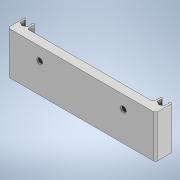
# Autodesk Inventor part: switch_mount
Saved by Autodesk Inventor 2020 (Build 240168000, 168)
## iProperties
Created: 2020-06-05
Part Number: switch_mount
Material: Generic
Document SubType Name: Modeling
Designer: suhren
Density: 1 g/cm^3
Appearance: Default
Author: suhren
Autodesk Inventor part; units mm, degrees
ref_plane "YZ Plane" through (0, 0, 0) normal (1, 0, 0) x (0, 1, 0)
ref_plane "XZ Plane" through (0, 0, 0) normal (0, 1, 0) x (-1, 0, 0)
ref_plane "XY Plane" through (0, 0, 0) normal (0, 0, 1) x (1, 0, 0)
sketch "Sketch1" plane through (0, 0, 0) normal (0, 1, 0) x (-1, 0, 0)
  line L0 (51.25, 0) -> (-51.25, 0)
  line L1 (-51.25, 0) -> (-51.25, 4.75)
  line L2 (-51.25, 6) -> (51.25, 6) construction
  line L3 (51.25, 6) -> (51.25, 4.75) construction
  line L4 (50, 6) -> (-50, 6)
  line L5 (-50, 6) -> (-51.25, 4.75)
  line L6 (50, 6) -> (51.25, 4.75)
  line L7 (51.25, 4.75) -> (51.25, 0)
  line L8 (-51.25, 4.75) -> (-51.25, 6) construction
  line L9 (47.5, -5.889) -> (44.95, -4.4167)
  line L10 (44.95, -4.4167) -> (44.95, -1.4722)
  line L11 (44.95, -1.4722) -> (47.5, 0)
  line L12 (47.5, 0) -> (50.05, -1.4722)
  line L13 (50.05, -1.4722) -> (50.05, -4.4167)
  line L14 (50.05, -4.4167) -> (47.5, -5.889)
  line L15 (47.5, -2.9445) -> (-47.5, -2.9445) construction
  line L16 (51.25, 0) -> (51.25, -5.0477)
  line L17 (51.25, -5.0477) -> (50.65, -5.6477)
  line L18 (50.65, -5.6477) -> (49.65, -4.6477)
  line L19 (50.05, -2.9445) -> (51.25, -2.9445) construction
  line L20 (45.35, -4.6477) -> (44.35, -5.6477)
  line L21 (44.35, -5.6477) -> (43.75, -5.0477)
  line L22 (43.75, -5.0477) -> (43.75, 0)
  line L23 (47.5, -5.889) -> (47.5, 0) construction
  line L24 (43.75, 0) -> (51.25, 0) construction
  point P0 (0, 0)
  point P1 (0, 0)
  point P2 (0, 0)
  point P3 (0, 6)
  point P4 (0, 6)
  point P5 (0, -2.9445)
  point P6 (50.65, -2.9445)
  dimension "d22" = 100
  dimension "d23" = 6
  dimension "d24" = 95
  dimension "d25" = 5.1
  dimension "d26" = 6
  dimension "d27" = 1.2
  dimension "d28" = 0.4
  constraints: 51 end point, 7 perpendicular, 7 point on line, 6 midpoint, 5 coincident, 5 parallel, 3 vertical, 2 horizontal, 2 horizontal alignment, 2 vertical alignment, 1 collinear, 16 other
  measures "d22" distance of L4.start L4.end
  measures "d23" distance between parallel lines of L0 L2
  measures "d24" distance of L15.end L15.start
  measures "d25" distance between parallel lines of L10 L13
  measures "d26" vertical distance of L2.end L11.end
  measures "d27" distance of L19.start L19.end
  measures "d28" horizontal distance of L18.end L13.end
extrude "Extrusion1" add sketch "Sketch1" along normal blind 29.5 contours L0 L1 L5 L4 L6 L7
extrude "Extrusion3" add sketch "Sketch1" along normal blind 29.5 contours L16 L17 L18 L14 L13 L12 L0 | L11 L10 L9 L20 L21 L22 L0
mirror "Mirror1" about plane through (0, 0, 0) normal (1, 0, 0) of "Extrusion3"
sketch "Sketch2" plane through (41.9, 0, 0) normal (0, 0, -1) x (-1, 0, 0)
  line L0 (41.9, 29.5) -> (41.9, 0) construction
  line L1 (12.9, 20.5) -> (70.9, 20.5) construction
  line L2 (9.35, 22.5496) -> (12.9, 24.5992)
  line L3 (12.9, 24.5992) -> (16.45, 22.5496)
  line L4 (16.45, 22.5496) -> (16.45, 18.4504)
  line L5 (16.45, 18.4504) -> (12.9, 16.4008)
  line L6 (12.9, 16.4008) -> (9.35, 18.4504)
  line L7 (9.35, 18.4504) -> (9.35, 22.5496)
  line L8 (74.45, 22.5496) -> (74.45, 18.4504)
  line L9 (74.45, 18.4504) -> (70.9, 16.4008)
  line L10 (70.9, 16.4008) -> (67.35, 18.4504)
  line L11 (67.35, 18.4504) -> (67.35, 22.5496)
  line L12 (67.35, 22.5496) -> (70.9, 24.5992)
  line L13 (70.9, 24.5992) -> (74.45, 22.5496)
  line L14 (-1.85, 0) -> (85.65, 0) construction
  line L15 (-1.85, 29.5) -> (85.65, 29.5) construction
  point P0 (41.9, 20.5)
  point P1 (41.9, 14.75)
  dimension "d9" = 58
  dimension "d10" = 7.1
  dimension "d34" = 9
  constraints: 28 end point, 3 midpoint, 3 vertical, 2 coincident, 1 horizontal, 1 parallel, 1 vertical alignment, 26 other
  measures "d9" distance of L1.start L1.end
  measures "d10" distance between parallel lines of L4 L7
  measures "d34" distance between parallel lines of L15 L1
extrude "Extrusion2" cut sketch "Sketch2" against normal blind 5
hole "Hole1" at (29, 20.5, 0) at (-29, 20.5, 0) direction (0, 0, 1) diameter 3.9 end through all
chamfer "Chamfer1" distance 1 angle 45 2 edges at (-43.75, 14.75, 0) (43.75, 14.75, 0)
body "Solid1"
